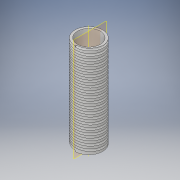
# Autodesk Inventor part: InnerThreadedPart
Saved by Autodesk Inventor 2019.2 (Build 232265000, 265)
## iProperties
Created: 2018-12-30
Part Number: InnerThreadedPart
Material: Generic
Document SubType Name: Modeling
Designer: steele
Density: 1 g/cm^3
Appearance: Default
Author: steele
Autodesk Inventor part; units mm, degrees
ref_plane "XZ Plane" through (0, 0, 0) normal (0, 1, 0) x (-1, 0, 0)
ref_plane "XY Plane" through (0, 0, 0) normal (0, 0, 1) x (1, 0, 0)
sketch "Sketch1" plane through (0, 0, 0) normal (0, 1, 0) x (-1, 0, 0)
  circle A0 centre (0, 0) radius 19.05
  circle A1 centre (0, 0) radius 15.875
  dimension "d4" = 31.75
  dimension "d5" = 38.1
  constraints: 2 centre point, 2 coincident
  measures "d4" diameter of A1
  measures "d5" diameter of A0
extrude "Extrusion1" add sketch "Sketch1" against normal blind 127
sketch "Sketch2" plane through (0, 0, 0) normal (1, 0, 0) x (0, 1, 0)
  line L0 (0, 19.05) -> (-127, 19.05) projected
  circle A0 centre (0, 19.05) radius 1.5875
  point P0 (0, 0)
  dimension "d18" = 3.175
  constraints: 1 centre point, 1 point on line
  measures "d18" diameter of A0
coil "Coil1" sketch "Sketch2" operation cut axis through (0, -10, 0) along (0, -1, 0) pitch 6.35 turns 20 hand left
sketch "Sketch4" plane through (0, -127, 0) normal (0, -1, 0) x (1, 0, 0)
  line L0 (-3.175, -17.1714) -> (-3.175, -22.225)
  line L1 (-3.175, -22.225) -> (3.175, -22.225)
  line L2 (3.175, -22.225) -> (3.175, -17.1714)
  line L3 (-3.175, -15.875) -> (3.175, -22.225) construction
  line L4 (-3.175, -22.225) -> (3.175, -15.875) construction
  arc A0 (-3.175, -17.1714) -> (3.175, -17.1714) centre (0, 0) ccw
  point P0 (0, -19.05)
  constraints: 10 end point, 2 midpoint, 2 point on circle, 1 centre point, 1 coincident, 1 parallel, 1 perpendicular, 1 vertical
extrude "Extrusion3" add sketch "Sketch4" against normal blind 50.8
body "Solid1"
